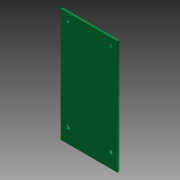
# Autodesk Inventor part: circuitBoard
Saved by Autodesk Inventor 2012 (Build 160160000, 160)
## iProperties
Created: 2013-12-16
Part Number: circuitBoard
Material: Default
Document SubType Name: Modeling
Designer: joe_000
Density: 1 g/cm^3
Author: joe_000
Autodesk Inventor part; units mm, degrees
ref_plane "YZ Plane" through (0, 0, 0) normal (1, 0, 0) x (0, 1, 0)
ref_plane "XZ Plane" through (0, 0, 0) normal (0, 1, 0) x (-1, 0, 0)
ref_plane "XY Plane" through (0, 0, 0) normal (0, 0, 1) x (1, 0, 0)
sketch "Sketch1" plane through (0, 0, 0) normal (0, 0, 1) x (1, 0, 0)
  line L0 (0, 0) -> (50.8, 0)
  line L1 (50.8, 0) -> (50.8, 101.6)
  line L2 (50.8, 101.6) -> (0, 101.6)
  line L3 (0, 101.6) -> (0, 0)
  dimension "d2" = 50.8
  dimension "d3" = 101.6
  constraints: 8 end point, 2 parallel, 1 horizontal, 1 perpendicular
  measures "d2" distance of L1.end L2.end
  measures "d3" distance of L0.end L1.end
extrude "Extrusion1" add sketch "Sketch1" along normal blind 1.6
sketch "Sketch2" plane through (0, 0, 1.6) normal (0, 0, 1) x (1, 0, 0)
  line L0 (0, 0) -> (0, 101.6) projected
  line L1 (50.8, 0) -> (0, 0) projected
  circle A0 centre (6.35, 12.7) radius 1.6383
  circle A1 centre (6.35, 95.25) radius 1.6383
  circle A2 centre (44.45, 12.7) radius 1.6383
  circle A3 centre (44.45, 95.25) radius 1.6383
  circle A4 centre (37.084, 87.376) radius 0.375
  line L2 (50.8, 101.6) -> (50.8, 0) projected
  circle A5 centre (39.624, 87.376) radius 0.375
  circle A6 centre (34.544, 87.376) radius 0.375
  dimension "d4" = 3.2766
  dimension "d7" = 82.55
  dimension "d10" = 38.1
  dimension "d13" = 6.35
  dimension "d14" = 12.7
  dimension "d17" = 0.75
  dimension "d20" = 87.376
  dimension "d21" = 13.716
  dimension "d22" = 2.54
  dimension "d23" = 2.54
  constraints: 7 centre point, 2 equal radius, 2 horizontal alignment, 1 horizontal, 1 vertical, 6 other
  measures "d4" diameter of A0
  measures "d7" distance of A0.centre A1.centre
  measures "d10" distance of A0.centre A2.centre
  measures "d13" distance from line of L0 A0.centre
  measures "d14" distance from line of L1 A0.centre
  measures "d17" diameter of A4
  measures "d20" distance from line of L1 A4.centre
  measures "d21" distance from line of L2 A4.centre
  measures "d22" distance of A4.centre A6.centre
  measures "d23" distance of A5.centre A4.centre
extrude "Extrusion2" cut sketch "Sketch2" against normal through all
body "Solid1"
